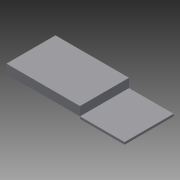
# Autodesk Inventor part: Robot sized box
Saved by Autodesk Inventor 2014 SP1 (Build 180222100, 222)
## iProperties
Created: 2014-01-25
Part Number: Robot sized box
Material: Generic
Document SubType Name: Modeling
Designer: Paul
Density: 1 g/cm^3
Appearance: Default
Author: Paul
Autodesk Inventor part; units mm, degrees
ref_plane "YZ Plane" through (0, 0, 0) normal (1, 0, 0) x (0, 1, 0)
ref_plane "XZ Plane" through (0, 0, 0) normal (0, 1, 0) x (-1, 0, 0)
ref_plane "XY Plane" through (0, 0, 0) normal (0, 0, 1) x (1, 0, 0)
sketch "Sketch1" plane through (0, 0, 0) normal (0, 0, 1) x (1, 0, 0)
  line L0 (-419.1, -50.8) -> (419.1, -50.8)
  line L1 (419.1, -50.8) -> (419.1, 50.8)
  line L2 (419.1, 50.8) -> (-419.1, 50.8)
  line L3 (-419.1, 50.8) -> (-419.1, -50.8)
  line L4 (-419.1, -50.8) -> (419.1, 50.8) construction
  line L5 (419.1, -50.8) -> (-419.1, 50.8) construction
  point P0 (0, 0)
  dimension "d0" = 838.2
  dimension "d1" = 101.6
  constraints: 12 end point, 2 midpoint, 2 parallel, 1 horizontal, 1 perpendicular
  measures "d0" distance of L2.end L1.end
  measures "d1" distance of L1.end L0.end
extrude "Extrusion1" add sketch "Sketch1" along normal blind 558.8
sketch "Sketch2" plane through (419.1, -50.8, 0) normal (1, 0, 0) x (0, 0, -1)
  line L0 (-558.8, 0) -> (0, 0)
  line L1 (0, 0) -> (0, -25.4)
  line L2 (0, -25.4) -> (-558.8, -25.4)
  line L3 (-558.8, -25.4) -> (-558.8, 0)
  point P0 (0, 50.8)
  dimension "d4" = 558.8
  dimension "d5" = 25.4
  constraints: 8 end point, 2 parallel, 1 horizontal, 1 perpendicular
  measures "d4" distance of L1.end L2.end
  measures "d5" distance of L0.end L1.end
extrude "Extrusion2" add sketch "Sketch2" along normal blind 508
body "Solid1"
